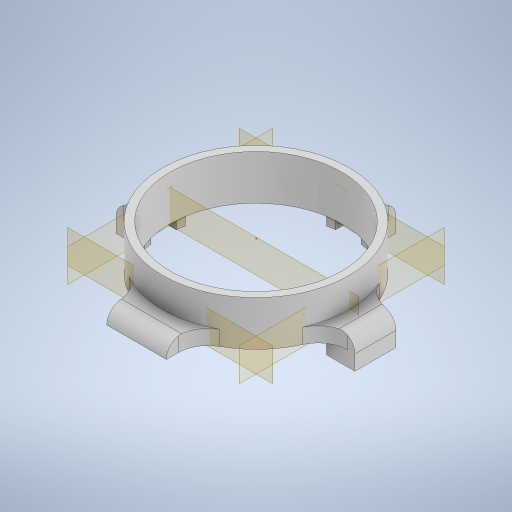
# Autodesk Inventor part: Widefield_Headplate_Adapter
Saved by Autodesk Inventor 2023 (Build 270158000, 158)
## iProperties
Created: 2023-02-09
Part Number: Widefield_Headplate_Adapter
Material: Generic
Document SubType Name: Modeling
Designer: User
Density: 1 g/cm^3
Appearance: Default
Author: User
Autodesk Inventor part; units mm, degrees
ref_plane "XZ Plane" through (0, 0, 0) normal (0, 1, 0) x (-1, 0, 0)
sketch "Sketch1" plane through (0, 0, 0) normal (0, 1, 0) x (-1, 0, 0)
  circle A0 centre (0, 0) radius 5.75
  circle A1 centre (0, 0) radius 6.25
  dimension "d0" = 11.5
  dimension "d1" = 12.5
  constraints: 2 centre point, 2 coincident
  measures "d0" diameter of A0
  measures "d1" diameter of A1
extrude "Extrusion1" add sketch "Sketch1" along normal blind 2
ref_plane "Work Plane1" through (0, 0, 5.75) normal (0, 0, 1) x (1, 0, 0)
ref_plane "Work Plane2" through (0, 0, -5.75) normal (0, 0, 1) x (1, 0, 0)
ref_plane "Work Plane3" through (5.75, 0, 0) normal (1, 0, 0) x (0, 1, 0)
ref_plane "Work Plane4" through (-5.75, 0, 0) normal (1, 0, 0) x (0, 1, 0)
sketch "Sketch4" plane through (0, 0, 5.75) normal (0, 0, 1) x (1, 0, 0)
  line L0 (6.25, 2) -> (-6.25, 2) projected
  line L1 (6.25, 0) -> (-6.25, 0) projected
  line L2 (-2, 2) -> (2, 2)
  line L3 (2, 2) -> (2, 0)
  line L4 (2, 0) -> (-2, 0)
  line L5 (-2, 0) -> (-2, 2)
  point P0 (0, 0)
  point P1 (0, 2)
  point P2 (-2, 0)
  dimension "d9" = 4
  dimension "d10" = 2
  constraints: 8 end point, 2 parallel, 2 point on line, 1 horizontal, 1 midpoint, 1 perpendicular
  measures "d9" distance between parallel lines of L3 L5
  measures "d10" distance from line of point (0, 2) L3
extrude "Extrusion3" add sketch "Sketch4" along normal blind 2.25
ref_plane "Work Plane5" through (0, 0, 0) normal (0, 0, 1) x (1, 0, 0)
sketch "Sketch6" plane through (-5.75, 0, 0) normal (1, 0, 0) x (0, 1, 0)
  line L0 (2, 5.75) -> (2, -5.75) projected
  line L1 (2, -1.375) -> (-1, -1.375)
  line L2 (-1, -1.375) -> (-1, 1.375)
  line L3 (-1, 1.375) -> (2, 1.375)
  line L4 (2, 1.375) -> (2, -1.375)
  line L5 (-2.6847, 0) -> (2.7808, 0) projected
  line L6 (0, -6.25) -> (0, 5.9214) projected
  point P0 (0, 0)
  point P1 (2, 1.375)
  dimension "d19" = 2.75
  dimension "d20" = 1.375
  dimension "d21" = 1
  constraints: 8 end point, 2 parallel, 1 horizontal, 1 perpendicular, 1 point on line
  measures "d19" distance of L1.end L2.end
  measures "d20" distance between parallel lines of L5 L3
  measures "d21" distance between parallel lines of L6 L2
extrude "Extrusion5" add sketch "Sketch6" against normal blind 2.25
sketch "Sketch7" plane through (-5.75, -1, -1.375) normal (0, -1, 0) x (1, 0, 0)
  line L0 (0, 2.75) -> (0, 0) projected
  line L1 (0, 0.525) -> (-1.7, 0.525)
  line L2 (-1.7, 0.525) -> (-1.7, 2.225)
  line L3 (-1.7, 2.225) -> (0, 2.225)
  line L4 (0, 2.225) -> (0, 0.525)
  line L5 (-5.1, 1.375) -> (14.85, 1.375) projected
  circle A0 centre (5.75, 1.375) radius 6.25
  circle A1 centre (5.75, 1.375) radius 5.75
  point P0 (-0.4419, 0.525)
  point P1 (-0.4419, 2.225)
  dimension "d24" = 1.7
  dimension "d25" = 1.7
  dimension "d26" = 0.85
  constraints: 8 end point, 2 centre point, 2 coincident, 2 parallel, 1 horizontal, 1 perpendicular, 1 point on line
  measures "d24" distance of L2.end L3.end
  measures "d25" distance of L1.end L2.end
  measures "d26" distance between parallel lines of L5 L3
extrude "Extrusion6" cut sketch "Sketch7" against normal blind 1
pattern_circular "Circular Pattern1" count 3 over 180 about axis through (0, 0, 0) along (0, -1, 0) of "Extrusion5", "Extrusion6"
sketch "Sketch8" plane through (0, 2, 0) normal (0, 1, 0) x (1, 0, 0)
  circle A0 centre (0, 0) radius 5.75
  circle A1 centre (0, 0) radius 5.75 projected
  circle A2 centre (0, 0) radius 8.6992
  constraints: 2 centre point, 2 coincident
extrude "Extrusion7" cut sketch "Sketch8" against normal blind 1
sketch "Sketch9" plane through (0, 1, 0) normal (0, 1, 0) x (1, 0, 0)
  circle A0 centre (0, 0) radius 5.75
  circle A1 centre (0, 0) radius 5.75 projected
  circle A2 centre (0, 0) radius 6.25
  constraints: 2 centre point, 2 coincident
extrude "Extrusion8" add sketch "Sketch9" along normal blind 2
fillet "Fillet1" radius 2 8 edges at (-6.0969, 0.5, -1.375) (-1.375, 0.5, -6.0969) (1.375, 0.5, -6.0969) (6.0969, 0.5, -1.375) (6.0969, 0.5, 1.375) (2, 0.5, 5.9214) (-2, 0.5, 5.9214) (-6.0969, 0.5, 1.375)
fillet "Fillet2" radius 1 4 edges at (-8, 1, 0) (0, 1, 8) (8, 1, 0) (0, 1, -8)
equation "\"d20\" = 0.5 * d19"
equation "\"d26\" = 0.5 * d25"
body "Solid1"
